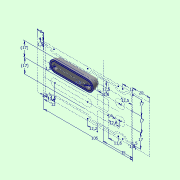
# Autodesk Inventor part: Large_retainer
Saved by Autodesk Inventor 2015 (Build 190159000, 159)
## iProperties
Created: 2015-06-18
Part Number: Large_retainer
Material: Generic
Document SubType Name: Modeling
Designer: Openlab
Density: 1 g/cm^3
Appearance: Default
Author: Openlab
Autodesk Inventor part; units mm, degrees
ref_plane "YZ Plane" through (0, 0, 0) normal (1, 0, 0) x (0, 1, 0)
ref_plane "XZ Plane" through (0, 0, 0) normal (0, 1, 0) x (-1, 0, 0)
ref_plane "XY Plane" through (0, 0, 0) normal (0, 0, 1) x (1, 0, 0)
sketch "Sketch1" plane through (0, 0, 0) normal (0, 1, 0) x (-1, 0, 0)
  line L0 (41.25, -2.25) -> (28.75, -2.25) construction
  line L1 (28.75, -2.25) -> (28.75, -14.75) construction
  line L2 (28.75, -14.75) -> (41.25, -14.75) construction
  line L3 (41.25, -14.75) -> (41.25, -2.25) construction
  line L4 (56.9183, -8.5) -> (8.3915, -8.5) construction
  line L5 (0, -17) -> (105, -17) construction
  line L6 (0, 0) -> (0, -51) construction
  line L7 (0, -34) -> (105, -34) construction
  line L8 (105, -51) -> (105, 0) construction
  line L9 (35, 19) -> (35, -51) construction
  line L10 (56.8064, -25.5) -> (17, -25.5) construction
  line L11 (28.75, -19.25) -> (28.75, -31.75) construction
  line L12 (41.25, -19.25) -> (28.75, -19.25) construction
  line L13 (41.25, -31.75) -> (41.25, -19.25) construction
  line L14 (28.75, -31.75) -> (41.25, -31.75) construction
  line L15 (28.75, -36.25) -> (28.75, -48.75) construction
  line L16 (41.25, -36.25) -> (28.75, -36.25) construction
  line L17 (41.25, -48.75) -> (41.25, -36.25) construction
  line L18 (28.75, -48.75) -> (41.25, -48.75) construction
  line L19 (56.3008, -42.5) -> (16.5498, -42.5) construction
  arc A0 (53.45, -12.2) -> (53.45, -21.8) centre (53.45, -17) ccw
  arc A1 (92, -21.8) -> (92, -12.2) centre (92, -17) ccw
  arc A2 (53.45, -29.2) -> (53.45, -38.8) centre (53.45, -34) ccw construction
  arc A3 (92, -38.8) -> (92, -29.2) centre (92, -34) ccw construction
  line L20 (53.45, -12.2) -> (92, -12.2)
  line L21 (53.45, -21.8) -> (92, -21.8)
  line L22 (53.45, -29.2) -> (92, -29.2) construction
  line L23 (53.45, -38.8) -> (92, -38.8) construction
  arc A4 (16.15, -38.6) -> (16.15, -29.4) centre (16.15, -34) ccw construction
  line L24 (103.5, -49.5) -> (103.5, -1.5) construction
  line L25 (1.5, -1.5) -> (1.5, -49.5) construction
  arc A5 (14, -29.4) -> (14, -38.6) centre (14, -34) ccw construction
  arc A6 (14, -12.4) -> (14, -21.6) centre (14, -17) ccw construction
  line L26 (16.15, -38.6) -> (14, -38.6) construction
  line L27 (14, -29.4) -> (16.15, -29.4) construction
  line L28 (14, -21.6) -> (16.15, -21.6) construction
  line L29 (16.15, -12.4) -> (14, -12.4) construction
  arc A7 (16.15, -21.6) -> (16.15, -12.4) centre (16.15, -17) ccw construction
  arc A8 (96.3, -51) -> (93, -47.7) centre (93, -51) ccw construction
  arc A9 (53.45, -47.7) -> (50.15, -51) centre (53.45, -51) ccw construction
  arc A10 (97.5596, -49.5) -> (93, -46.2) centre (93, -51) ccw construction
  line L30 (93, -46.2) -> (53.45, -46.2) construction
  line L31 (96.3, -51) -> (105, -51) construction
  line L32 (93, -47.7) -> (53.45, -47.7) construction
  line L33 (105, -49.5) -> (97.5596, -49.5) construction
  arc A11 (53.45, -46.2) -> (48.8904, -49.5) centre (53.45, -51) ccw construction
  arc A12 (48.8904, -1.5) -> (53.45, -4.8) centre (53.45, 0) ccw construction
  arc A13 (50.15, 0) -> (53.45, -3.3) centre (53.45, 0) ccw construction
  line L34 (93, -3.3) -> (53.45, -3.3) construction
  line L35 (93, -4.8) -> (53.45, -4.8) construction
  line L36 (97.5596, -1.5) -> (105, -1.5) construction
  line L37 (105, 0) -> (96.3, 0) construction
  arc A14 (93, -3.3) -> (96.3, 0) centre (93, 0) ccw construction
  arc A15 (93, -4.8) -> (97.5596, -1.5) centre (93, 0) ccw construction
  arc A16 (20.45, -51) -> (17.15, -47.7) centre (17.15, -51) ccw construction
  arc A17 (12, -47.7) -> (8.7, -51) centre (12, -51) ccw construction
  line L38 (17.15, -46.2) -> (12, -46.2) construction
  line L39 (17.15, -47.7) -> (12, -47.7) construction
  arc A18 (12, -46.2) -> (7.4404, -49.5) centre (12, -51) ccw construction
  arc A19 (21.7096, -49.5) -> (17.15, -46.2) centre (17.15, -51) ccw construction
  line L40 (48.8904, -49.5) -> (21.7096, -49.5) construction
  line L41 (7.4404, -49.5) -> (0, -49.5) construction
  line L42 (0, -51) -> (8.7, -51) construction
  line L43 (20.45, -51) -> (50.15, -51) construction
  line L44 (17.15, -4.8) -> (12, -4.8) construction
  line L45 (17.15, -3.3) -> (12, -3.3) construction
  arc A20 (8.7, 0) -> (12, -3.3) centre (12, 0) ccw construction
  arc A21 (17.15, -3.3) -> (20.45, 0) centre (17.15, 0) ccw construction
  arc A22 (7.4404, -1.5) -> (12, -4.8) centre (12, 0) ccw construction
  arc A23 (17.15, -4.8) -> (21.7096, -1.5) centre (17.15, 0) ccw construction
  line L46 (50.15, 0) -> (20.45, 0) construction
  line L47 (8.7, 0) -> (0, 0) construction
  line L48 (0, -1.5) -> (7.4404, -1.5) construction
  line L49 (21.7096, -1.5) -> (48.8904, -1.5) construction
  line L50 (113, 2) -> (-20, 2) construction
  line L51 (-20, 2) -> (-20, -53) construction
  line L52 (-20, -53) -> (113, -53) construction
  line L53 (113, -53) -> (113, 2) construction
  arc A24 (92, -23.3) -> (92, -10.7) centre (92, -17) ccw
  arc A25 (53.45, -10.7) -> (53.45, -23.3) centre (53.45, -17) ccw
  line L54 (92, -10.7) -> (53.45, -10.7)
  line L55 (53.45, -23.3) -> (92, -23.3)
  point P0 (35, -8.5)
  point P1 (35, -42.5)
  point P2 (35, -25.5)
  dimension "d0" = 12.5
  dimension "d1" = 12.5
  dimension "d2" = 17
  dimension "d3" = 35
  dimension "d4" = 105
  dimension "d5" = 17
  dimension "d6" = 17
  dimension "d7" = 9.6
  dimension "d8" = 1.5
  dimension "d9" = 1.5
  dimension "d10" = 4.6
  dimension "d11" = 1.5
  dimension "d12" = 1.5
  dimension "d13" = 1.5
  dimension "d14" = 17
  dimension "d15" = 17
  dimension "d16" = 12
  dimension "d17" = 13
  dimension "d18" = 12.2
  dimension "d19" = 11.6
  dimension "d20" = 12.6
  dimension "d21" = 12
  dimension "d22" = 12.5
  dimension "d23" = 2
  dimension "d24" = 8
  dimension "d25" = 20
  dimension "d26" = 1.5
  constraints: 112 end point, 52 point on circle, 28 point on line, 28 tangent, 26 centre point, 22 equal radius, 16 coincident, 16 parallel, 15 perpendicular, 14 horizontal, 13 collinear, 9 vertical alignment, 7 horizontal alignment, 1 vertical, 9 other
  measures "d0" distance of L2.end L1.end
  measures "d1" distance of L0.end L1.end
  measures "d2" distance between parallel lines of L10 L4
  measures "d3" distance between parallel lines of L6 L9
  measures "d4" distance between parallel lines of L6 L8
  measures "d5" distance between parallel lines of L19 L10
  measures "d6" distance between parallel lines of L5 L7
  measures "d7" diameter of A0
  measures "d8" distance between parallel lines of L6 L25
  measures "d9" distance between parallel lines of L8 L24
  measures "d10" radius of A4
  measures "d11" radial gap between concentric circles of A8 A10
  measures "d12" distance between parallel lines of L37 L36
  measures "d13" distance between parallel lines of L41 L42
  measures "d14" distance between parallel lines of L7 L42
  measures "d15" distance between parallel lines of L47 L5
  measures "d16" distance from line of A8.centre L8
  measures "d17" distance from line of L8 A3.centre
  measures "d18" distance from line of A9.centre L17
  measures "d19" distance from line of A19.centre L15
  measures "d20" distance from line of A4.centre L15
  measures "d21" distance from line of L6 A22.centre
  measures "d22" distance from line of L25 A6.centre
  measures "d23" distance between parallel lines of L50 L37
  measures "d24" distance between parallel lines of L8 L53
  measures "d25" distance between parallel lines of L51 L6
  measures "d26" radial gap between concentric circles of A24 A1
extrude "Extrusion1" add sketch "Sketch1" along normal blind 8.5 contours L20 A1 L21 A0
extrude "Extrusion2" add sketch "Sketch1" along normal blind 4
chamfer "Chamfer1" distance 0.5 angle 45 4 edges at (-72.725, 8.5, -12.2) (-48.65, 8.5, -17) (-72.725, 8.5, -21.8) (-96.8, 8.5, -17)
hole "Hole1" at (-35, 0, -8.5) at (0, 0, -17) at (-35, 0, -42.5) at (-35, 0, -25.5) at (-92, 0, -17) at (-53.45, 0, -17) direction (0, 1, 0) diameter 4 end through all counterbore diameter 6 counterbore depth 3
body "Solid1"
